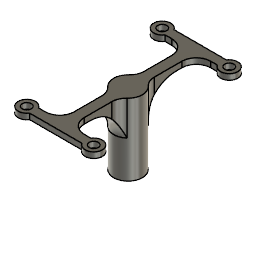
Baugruppe Tank ohne Ketten (Autodesk Fusion 360 archive; units mm, degrees)
design "ESP32 Halter"
Autodesk Fusion 360 part; units mm, degrees
sketch "Skizze1" plane through (0, 0, 0) normal (0, 0, 1) x (1, 0, 0)
  line L0 (0, 53) -> (30, 53)
  line L1 (30, 53) -> (30, 0)
  line L2 (30, 0) -> (0, 0)
  line L3 (0, 0) -> (0, 53)
  circle A0 centre (3.35, 50.05) radius 1.575
  circle A1 centre (26.65, 50.05) radius 1.575
  circle A2 centre (26.65, 2.95) radius 1.575
  circle A3 centre (3.35, 2.95) radius 1.575
  circle A4 centre (3.35, 50.05) radius 3
  circle A5 centre (3.35, 2.95) radius 3
  circle A6 centre (26.65, 2.95) radius 3
  circle A7 centre (26.65, 50.05) radius 3
  line L4 (25.2383, 2.2516) -> (1.9383, 49.3516)
  line L5 (28.0617, 3.6484) -> (4.7617, 50.7484)
  line L6 (25.2383, 50.7484) -> (1.9383, 3.6484)
  line L7 (4.7617, 2.2516) -> (28.0617, 49.3516)
  line L8 (15, 22.9479) -> (15, 30.0521)
  line L9 (16.7572, 26.5) -> (13.2428, 26.5)
  circle A8 centre (15, 26.5) radius 5
  line L10 (26.7145, 1.3763) -> (3.2412, 1.3763)
  line L11 (3.2412, 1.3763) -> (3.2412, 4.5212)
  line L12 (3.2412, 4.5212) -> (26.7145, 4.5212)
  line L13 (26.7145, 4.5212) -> (26.7145, 1.3763)
  line L14 (13.2428, 26.5) -> (16.7572, 26.5)
  line L15 (16.7572, 26.5) -> (16.7572, 1.3763)
  line L16 (16.7572, 1.3763) -> (13.2428, 1.3763)
  line L17 (13.2428, 1.3763) -> (13.2428, 26.5)
  line L18 (3.444, 51.6222) -> (26.65, 51.6222)
  line L19 (26.65, 51.6222) -> (26.65, 48.475)
  line L20 (26.65, 48.475) -> (3.444, 48.475)
  line L21 (3.444, 48.475) -> (3.444, 51.6222)
  line L22 (16.7572, 26.5) -> (13.2428, 26.5)
  line L23 (13.2428, 26.5) -> (13.2428, 51.6222)
  line L24 (13.2428, 51.6222) -> (16.7572, 51.6222)
  line L25 (16.7572, 51.6222) -> (16.7572, 26.5)
  dimension "d1" = 30
  dimension "d2" = 53
  dimension "d9" = 3.15
  dimension "d10" = 47.1
  dimension "d11" = 23.3
  dimension "d14" = 6
  dimension "d15" = 3.35
  dimension "d18" = 2.95
  dimension "d19" = 10
  constraint horizontal L0
  constraint vertical L1
  constraint horizontal L2
  constraint vertical L3
  constraint coincident L2.end L3.start
  constraint horizontal A0.centre A1.centre
  constraint vertical A1.centre A2.centre
  constraint horizontal A2.centre A3.centre
  constraint vertical A0.centre A3.centre
  constraint equal A0 A1
  constraint equal A0 A3
  constraint equal A0 A2
  constraint concentric A0 A4
  constraint equal A4 A7
  constraint equal A4 A5
  constraint equal A4 A6
  constraint vertical A2.centre A1.centre
  constraint horizontal A3.centre A2.centre
  constraint coincident A1.centre A7.centre
  constraint coincident A2.centre A6.centre
  constraint coincident A2 L4.start
  constraint coincident A0 L4.end
  constraint tangent A0 L4
  constraint tangent A2 L4
  constraint coincident A2 L5.start
  constraint coincident A0 L5.end
  constraint tangent A0 L5
  constraint coincident A1 L6.start
  constraint coincident A3 L6.end
  constraint tangent A3 L6
  constraint coincident A3 L7.start
  constraint coincident A1 L7.end
  constraint tangent A1 L7
  constraint tangent A1 L6
  constraint tangent A3 L7
  constraint tangent A2 L5
  constraint coincident L7 L8.start
  constraint coincident L4 L8.start
  constraint coincident L5 L8.end
  constraint coincident L6 L8.end
  constraint coincident L5 L9.start
  constraint coincident L7 L9.start
  constraint coincident L4 L9.end
  constraint coincident L6 L9.end
  constraint coincident L8 A8.centre
  constraint coincident L9 A8.centre
  constraint horizontal L10
  constraint vertical L11
  constraint horizontal L12
  constraint vertical L13
  constraint coincident A3 L11.end
  constraint coincident A2 L10.start
  constraint horizontal L14
  constraint vertical L15
  constraint horizontal L16
  constraint vertical L17
  constraint coincident L10 L15.end
  constraint coincident L9.start L15
  constraint horizontal L18
  constraint vertical L19
  constraint horizontal L20
  constraint vertical L21
  constraint coincident A1 L19.end
  constraint coincident A0 L18.start
  constraint horizontal L22
  constraint vertical L23
  constraint horizontal L24
  constraint vertical L25
  constraint coincident L18 L23.end
  measures "d1" distance of L0.start L0.end
  measures "d2" distance of L0.start L2.end
  measures "d9" diameter of A0
  measures "d10" distance of A0.centre A3.centre
  measures "d11" distance of A0.centre A1.centre
  measures "d14" diameter of A4
  measures "d15" distance of L3 A0.centre
  measures "d18" distance of L0 A0.centre
  measures "d19" diameter of A8
extrude "Extrusion1" add sketch "Skizze1" along normal blind 2 contours L0 A4 | L0 A0 A4 L4 L18 | A0 A4 L4 L5 L20 L21 | L2 A3 A5 L6 L10 L11 | L2 A5 | L0 A7 | L0 A1 A7 L7 L18 | A4 L18 L20 L23 | A0 A4 L5 L18 L20 | A4 L5 L20 | L4 A8 L23 | L4 L6 A8 | A3 L7 L12 | A3 A5 L6 L7 L12 | A1 A7 L6 L18 L20 | A7 L18 L20 L25 | L18 L20 L23 L24 L25 | L5 L6 A8 L20 L23 L25 | L5 A8 L23 | A0 L5 L20 L21 | L4 L8 L9 L14 L22 | L5 L6 A8 L23 | L6 A8 L17 | L6 L8 L9 L14 L22 | L4 L7 A8 L17 | A2 A6 L4 L10 L12 | L2 A2 A6 L5 L10 | L2 A6 | A3 A5 L7 L10 L12 | A5 L10 L12 L17 | A5 L7 L12 | A7 L6 L20 | L5 L6 A8 | L4 L7 A8 L15 | L7 L8 L9 L14 L22 | L4 L7 A8 | L5 L6 A8 L25 | L5 L8 L9 L14 L22 | L7 A8 L17 | A6 L10 L12 L15 | L10 L12 L15 L16 L17 | L4 L7 A8 L12 L15 L17 | A1 A7 L6 L7 L20 | A1 L6 L20 | L6 A8 L25 | L4 A8 L15 | L5 L7 A8 | L7 A8 L25 | L5 A8 L15 | A6 L4 L12 | A2 A6 L4 L5 L12 | A2 L4 L12
extrude "Extrusion4" add sketch "Skizze1" against normal blind 23 contours L4 A8 L23 | L4 L6 A8 | L4 L8 L9 L14 L22 | L5 L6 A8 L23 | L6 A8 L17 | L6 L8 L9 L14 L22 | L4 L7 A8 L17 | L5 L6 A8 | L4 L7 A8 L15 | L7 L8 L9 L14 L22 | L4 L7 A8 | L5 L6 A8 L25 | L5 L8 L9 L14 L22 | L5 L7 A8 | L7 A8 L25 | L5 A8 L15
extrude "Extrusion6" add sketch "Skizze1" along normal blind 2 contours L0 A4 | L0 A0 A4 L4 L18 | A0 A4 L4 L5 L20 L21 | L2 A3 A5 L6 L10 L11 | L2 A5 | L0 A7 | L0 A1 A7 L7 L18 | A0 A4 L5 L18 L20 | A4 L5 L20 | A3 L7 L12 | A3 A5 L6 L7 L12 | A1 A7 L6 L18 L20 | A0 L5 L20 L21 | A2 A6 L4 L10 L12 | L2 A2 A6 L5 L10 | L2 A6 | A3 A5 L7 L10 L12 | A5 L7 L12 | A7 L6 L20 | A1 A7 L6 L7 L20 | A1 L6 L20 | A6 L4 L12 | A2 A6 L4 L5 L12 | A2 L4 L12
hole "Bohrung1" at (15, 26.5, -23) direction (0, 0, 1) diameter 3.2 depth 8 tip angle 118
move_face "Flächen versetzen1" [suppressed]
ref_plane "Arbeitsebene1" through (6.3686, 5.5, 1) normal (-0.443071, -0.896486, 0) x (0, 0, 1)
sketch "Skizze2" plane through (3.4349, 6.95, 0) normal (-0.443071, -0.896486, 0) x (0, 0, 1)
  line L0 (0, -3.2797) -> (2, -3.2797)
  line L1 (12.5, -3.446) -> (12.5, -28)
  line L2 (12.5, -28) -> (0, -28)
  line L3 (0, -28) -> (0, -3.446)
  line L4 (0, -3.446) -> (12.5, -3.446)
  constraint vertical L1
  constraint horizontal L2
  constraint vertical L3
  constraint perpendicular L1 L4
  constraint coincident L1 L4.end
  constraint coincident L1.start L4.end
extrude "Extrusion5" [suppressed]
fillet "Abrundung2" radius 5 8 edges at (13.2428, 4.5212, 1) (16.7572, 4.5212, 1) (16.7572, 48.475, 1) (13.2428, 48.475, 1) (13.2428, 31.1811, 1) (13.2428, 21.8189, 1) (16.7572, 21.8189, 1) (16.7572, 31.1811, 1)
fillet "Abrundung3" radius 10 2 edges at (15, 31.5, 0) (15, 21.5, 0)
equation "d10 = 43.8 mm + 3.3 mm"
equation "d11 = 20 mm + 3.3 mm"
equation "d15 = ( d1 - d11 ) / 2"
equation "d18 = ( d2 - d10 ) / 2"
equation "d30 = 63.7 deg + 90 deg"

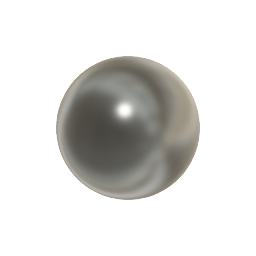
design "Kugel für Kugelhalter"
Autodesk Fusion 360 part; units mm, degrees
sketch "Skizze1" plane through (0, 0, 0) normal (0, 1, 0) x (1, 0, 0)
  line L0 (0, -5.95) -> (0, 5.95)
  arc A0 (0, -5.95) -> (0, 5.95) centre (0, 0) ccw
  dimension "d1" = 11.9
  constraint coincident A0.centre origin
  constraint vertical L0
  measures "d1" diameter of A0
revolve "Drehen1" add sketch "Skizze1" angle 360 about axis through (0, 0, 5.95) along (0, 0, -1)

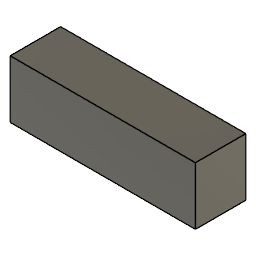
design "Batteriekörper"
Autodesk Fusion 360 part; units mm, degrees
sketch "Skizze1" plane through (0, 0, 0) normal (0, 0, 1) x (1, 0, 0)
  line L0 (38.5, -10.5) -> (-38.5, -10.5)
  line L1 (-38.5, -10.5) -> (-38.5, 10.5)
  line L2 (-38.5, 10.5) -> (38.5, 10.5)
  line L3 (38.5, 10.5) -> (38.5, -10.5)
  circle A0 centre (28.5, 0) radius 1.25
  circle A1 centre (-28.5, 0) radius 1.25
  point P0 (29.4587, 0)
  dimension "d1" = 77
  dimension "d2" = 21
  dimension "d5" = 2.5
  dimension "d6" = 10
  dimension "d7" = 10.5
  dimension "d8" = 2.5
  dimension "d9" = 10
  dimension "d13" = 57
  dimension "d14" = 38.5
  constraint horizontal L0
  constraint vertical L1
  constraint horizontal L2
  constraint vertical L3
  constraint horizontal A0.centre A1.centre
  constraint horizontal origin A1.centre
  measures "d1" distance of L0.start L0.end
  measures "d2" distance of L0.start L2.end
  measures "d5" diameter of A0
  measures "d6" distance of L3 A0.centre
  measures "d7" vertical distance of L0.start A0.centre
  measures "d8" diameter of A1
  measures "d9" distance of L1 A1.centre
  measures "d13" horizontal distance of A0.centre A1.centre
  measures "d14" distance of origin L3
extrude "Extrusion1" add sketch "Skizze1" along normal blind 24 contours L0 L1 L2 L3 | A0 | A1
extrude "Extrusion2" cut sketch "Skizze1" along normal blind 5 contours A0 | A1
equation "d7 = d2 / 2"
equation "d14 = d1 / 2"

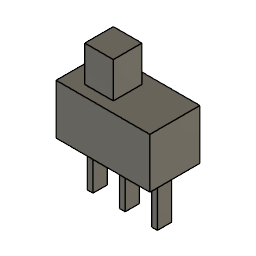
design "Schalter"
Autodesk Fusion 360 part; units mm, degrees
sketch "Skizze1" plane through (0, 0, 0) normal (0, 0, 1) x (1, 0, 0)
  line L0 (0, 7) -> (13.1, 7)
  line L1 (13.1, 7) -> (13.1, 0)
  line L2 (13.1, 0) -> (0, 0)
  line L3 (0, 0) -> (0, 7)
  dimension "d1" = 13.1
  dimension "d2" = 7
  constraint horizontal L0
  constraint vertical L1
  constraint horizontal L2
  constraint vertical L3
  constraint coincident L2.end L3.start
  measures "d1" distance of L0.start L0.end
  measures "d2" distance of L0.start L2.end
extrude "Extrusion1" add sketch "Skizze1" along normal blind 7
sketch "Skizze2" plane through (0, 0, 7) normal (0, 0, 1) x (-1, 0, 0)
  line L0 (0, 0) -> (-13.1, 0)
  line L1 (-13.1, 0) -> (-13.1, -7)
  line L2 (-13.1, -7) -> (0, -7)
  line L3 (0, -7) -> (0, 0)
  line L4 (-2.5, -5.5) -> (-6.5, -5.5)
  line L5 (-6.5, -5.5) -> (-6.5, -1.5)
  line L6 (-6.5, -1.5) -> (-2.5, -1.5)
  line L7 (-2.5, -1.5) -> (-2.5, -5.5)
  dimension "d5" = 4
  dimension "d6" = 4
  constraint horizontal L4
  constraint vertical L5
  constraint horizontal L6
  constraint vertical L7
  measures "d5" distance of L4.start L4.end
  measures "d6" distance of L4.start L6.end
extrude "Extrusion2" add sketch "Skizze2" along normal blind 5 contours L4 L5 L6 L7
sketch "Skizze3" plane through (0, 0, 0) normal (0, 0, -1) x (1, 0, 0)
  line L0 (13.1, 0) -> (0, 0)
  line L1 (0, 0) -> (0, -7)
  line L2 (0, -7) -> (13.1, -7)
  line L3 (13.1, -7) -> (13.1, 0)
  line L4 (10.9487, -2.4048) -> (11.7487, -2.4048)
  line L5 (11.7487, -2.4048) -> (11.7487, -4.4048)
  line L6 (11.7487, -4.4048) -> (10.9487, -4.4048)
  line L7 (10.9487, -4.4048) -> (10.9487, -2.4048)
  line L8 (6.4487, -2.4048) -> (7.2487, -2.4048)
  line L9 (7.2487, -2.4048) -> (7.2487, -4.4048)
  line L10 (6.4487, -4.4048) -> (6.4487, -2.4048)
  line L11 (7.2487, -4.4048) -> (6.4487, -4.4048)
  line L12 (1.9487, -2.4048) -> (2.7487, -2.4048)
  line L13 (2.7487, -2.4048) -> (2.7487, -4.4048)
  line L14 (1.9487, -4.4048) -> (1.9487, -2.4048)
  line L15 (2.7487, -4.4048) -> (1.9487, -4.4048)
  dimension "d9" = 0.8
  dimension "d10" = 2
  dimension "d13" = -9
  dimension "d14" = 0
  constraint horizontal L4
  constraint vertical L5
  constraint horizontal L6
  constraint vertical L7
  measures "d9" distance of L4.start L4.end
  measures "d10" distance of L4.start L6.end
extrude "Extrusion3" add sketch "Skizze3" along normal blind 6.5 contours L4 L5 L6 L7 | L8 L9 L10 L11 | L12 L13 L14 L15

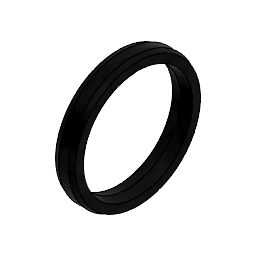
design "Reifen"
Autodesk Fusion 360 part; units mm, degrees
sketch "Skizze1" plane through (0, 0, 0) normal (0, 0, 1) x (1, 0, 0)
  line L0 (10, -22.5) -> (10, -27.5)
  line L1 (10, -22.5) -> (0, -22.5)
  arc A0 (0, -27.5) -> (10, -27.5) centre (5, -27.5) ccw
  line L2 (0, -22.5) -> (0, -27.5)
  line L3 (0, -27.5) -> (5, -26.5)
  line L4 (5, -26.5) -> (10, -27.5)
  line L5 (2.5, -32.5) -> (7.5, -32.5)
  line L6 (2.5, -32.5) -> (0, -31.5)
  line L7 (0, -31.5) -> (0, -27.5)
  line L8 (7.5, -32.5) -> (10, -31.5)
  line L9 (10, -31.5) -> (10, -27.5)
  dimension "d1" = 5
  dimension "d2" = 27.5
  dimension "d3" = 5
  dimension "d5" = 1
  dimension "d7" = 5
  dimension "d8" = 4
  constraint horizontal L1
  constraint perpendicular L1 L2
  constraint perpendicular L0 L1
  constraint equal L0 L2
  constraint vertical L1.end origin
  constraint horizontal L0.end A0.centre
  constraint vertical A0.centre L3.end
  constraint horizontal L5
  constraint tangent A0 L7
  constraint tangent A0 L9
  constraint horizontal L6.end L8.end
  constraint tangent A0 L5
  constraint equal L6 L8
  measures "d1" radius of A0
  measures "d2" vertical distance of A0.centre origin
  measures "d3" distance of L0.end L0.start
  measures "d5" distance of A0.centre L3.end
  measures "d7" distance of L5.start L5.end
  measures "d8" distance of A0.start L6.end
revolve "Drehen1" add sketch "Skizze1" angle 360 about axis through (1.75, 0, 0) along (1, 0, 0) contours A0 L5 L8 L9 | A0 L3 L4 | A0 L5 L6 L7
sketch "Skizze2" plane through (0, 0, 0) normal (0, 1, 0) x (1, 0, 0)
  line L0 (0, -28.6) -> (10, -28.6)
  line L1 (10, -28.6) -> (10, -26.4)
  line L2 (10, -26.4) -> (0, -26.4)
  line L3 (0, -26.4) -> (0, -28.6)
  line L4 (2.5, 32.5) -> (2.5, -32.5)
  line L5 (0, 31.5) -> (0, -31.5)
  line L6 (10, 31.5) -> (10, -31.5)
  line L7 (7.5, 32.5) -> (7.5, -32.5)
  line L8 (9, -28.6) -> (10, -27.6)
  line L9 (1, -28.6) -> (0, -27.6)
  dimension "d9" = 2.2
  dimension "d10" = 26.4
  dimension "d15" = 45
  dimension "d16" = 1
  dimension "d17" = 45
  constraint horizontal L0
  constraint vertical L1
  constraint horizontal L2
  constraint vertical L3
  constraint coincident L0.start L5
  constraint coincident L0.end L6
  constraint coincident L0 L8.start
  constraint coincident L6 L8.end
  constraint coincident L0 L9.start
  constraint coincident L5 L9.end
  constraint equal L8 L9
  measures "d9" distance of L0.start L2.end
  measures "d10" distance of origin L2
  measures "d15" angle of L1 L8
  measures "d16" distance of L0.end L8.end
  measures "d17" angle of L3 L9
extrude "Extrusion1" cut sketch "Skizze2" along normal mid plane 2.3 contours L0 L2 L3 L4 L5 L9 | L0 L2 L4 L7 | L0 L1 L2 L6 L7 L8

design "Servomotor Antrieb STS3215"
Autodesk Fusion 360 part; units mm, degrees
sketch "Skizze1" plane through (0, 0, 0) normal (0, 0, 1) x (1, 0, 0)
  line L0 (0, 45.5) -> (35, 45.5)
  line L1 (35, 45.5) -> (35, 0)
  line L2 (35, 0) -> (0, 0)
  line L3 (0, 0) -> (0, 45.5)
  line L4 (35, 45.5) -> (35, 25.5)
  dimension "d1" = 35
  dimension "d2" = 45.5
  constraint horizontal L0
  constraint vertical L1
  constraint horizontal L2
  constraint vertical L3
  constraint coincident L2.end L3.start
  constraint vertical L4
  constraint collinear L1 L4
  measures "d1" distance of L0.start L0.end
  measures "d2" distance of L0.end L1.end
extrude "Extrusion4" add sketch "Skizze1" along normal blind 25
sketch "Skizze4" plane through (35, 0, 0) normal (1, 0, 0) x (0, 1, 0)
  line L0 (0, 0) -> (45.5, 0)
  line L1 (45.5, 0) -> (45.5, 25)
  line L2 (45.5, 25) -> (0, 25)
  line L3 (0, 25) -> (0, 0)
  circle A0 centre (10, 12.5) radius 10
  dimension "d29" = 20
  dimension "d30" = 12.5
  constraint tangent L3 A0
  measures "d29" diameter of A0
  measures "d30" distance of L0 A0.centre
extrude "Extrusion5" add sketch "Skizze4" along normal blind 1.6 contours A0
equation "d30 = ( 25 / 2 ) * 1 mm"
